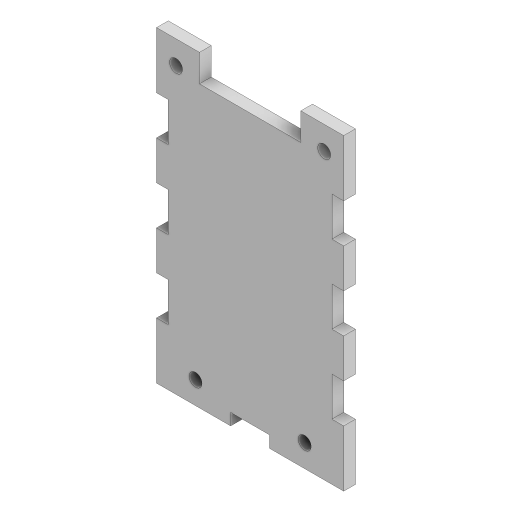
# Autodesk Inventor part: Bottom piece
Saved by Autodesk Inventor 2023.3 (Build 273359000, 359)
## iProperties
Created: 2024-09-20
Part Number: Bottom piece
Material: Generic
Document SubType Name: Modeling
Designer: David Zindović
Density: 1 g/cm^3
Appearance: Default
Author: David Zindović
Autodesk Inventor part; units mm, degrees
ref_plane "YZ Plane" through (0, 0, 0) normal (1, 0, 0) x (0, 1, 0)
ref_plane "XZ Plane" through (0, 0, 0) normal (0, 1, 0) x (-1, 0, 0)
ref_plane "XY Plane" through (0, 0, 0) normal (0, 0, 1) x (1, 0, 0)
sketch "Sketch1" plane through (0, 0, 0) normal (0, 0, 1) x (1, 0, 0)
  circle A0 centre (-22.4743, -28.7795) radius 1.65
  circle A1 centre (5.5257, -28.7795) radius 1.65
  circle A2 centre (-27.4743, 38.4705) radius 1.65
  circle A3 centre (10.5257, 38.4705) radius 1.65
  line L0 (-25.4743, 18.4705) -> (8.5257, 18.4705)
  line L1 (8.5257, 18.4705) -> (8.5257, -25.5295)
  line L2 (8.5257, -25.5295) -> (-25.4743, -25.5295)
  line L3 (-25.4743, -25.5295) -> (-25.4743, 18.4705)
  circle A4 centre (-8.4743, 28.4705) radius 2.5
  line L4 (-32.4743, 44.4705) -> (15.5257, 44.4705)
  line L5 (15.5257, 44.4705) -> (15.5257, -34.5295)
  line L6 (15.5257, -34.5295) -> (-32.4743, -34.5295)
  line L7 (-32.4743, -34.5295) -> (-32.4743, 44.4705)
  line L8 (-25.4743, -25.5295) -> (8.5257, -25.5295)
  line L9 (8.5257, -25.5295) -> (8.5257, -26.5295)
  line L10 (8.5257, -26.5295) -> (-25.4743, -26.5295)
  line L11 (-25.4743, -26.5295) -> (-25.4743, -25.5295)
  line L12 (-24.1243, -28.7795) -> (-24.1243, -26.5295)
  line L13 (-20.8243, -28.7795) -> (-20.8243, -26.5295)
  line L14 (3.8757, -28.7795) -> (3.8757, -26.5295)
  line L15 (7.1757, -28.7795) -> (7.1757, -26.5295)
  line L16 (-32.4743, 9.9705) -> (-29.4743, 9.9705)
  line L17 (-29.4743, 9.9705) -> (-29.4743, -0.0295)
  line L18 (-29.4743, -0.0295) -> (-32.4743, -0.0295)
  line L19 (-32.4743, -0.0295) -> (-32.4743, 9.9705)
  line L20 (-13.4743, -34.5295) -> (-3.4743, -34.5295)
  line L21 (-3.4743, -34.5295) -> (-3.4743, -31.5295)
  line L22 (-3.4743, -31.5295) -> (-13.4743, -31.5295)
  line L23 (-13.4743, -31.5295) -> (-13.4743, -34.5295)
  line L24 (-13.4743, 44.4705) -> (-3.4743, 44.4705)
  line L25 (-3.4743, 44.4705) -> (-3.4743, 41.4705)
  line L26 (-3.4743, 41.4705) -> (-13.4743, 41.4705)
  line L27 (-13.4743, 41.4705) -> (-13.4743, 44.4705)
  line L28 (-29.4743, 29.9705) -> (-29.4743, 19.9705)
  line L29 (-29.4743, 19.9705) -> (-32.4743, 19.9705)
  line L30 (-32.4743, 29.9705) -> (-29.4743, 29.9705)
  line L31 (-29.4743, -20.0295) -> (-32.4743, -20.0295)
  line L32 (-29.4743, -10.0295) -> (-29.4743, -20.0295)
  line L33 (-32.4743, -10.0295) -> (-29.4743, -10.0295)
  line L34 (12.5257, 9.9705) -> (15.5257, 9.9705)
  line L35 (15.5257, 9.9705) -> (15.5257, -0.0295)
  line L36 (15.5257, -0.0295) -> (12.5257, -0.0295)
  line L37 (12.5257, -0.0295) -> (12.5257, 9.9705)
  line L38 (15.5257, -20.0295) -> (12.5257, -20.0295)
  line L39 (12.5257, -20.0295) -> (12.5257, -10.0295)
  line L40 (12.5257, -10.0295) -> (15.5257, -10.0295)
  line L41 (15.5257, 19.9705) -> (12.5257, 19.9705)
  line L42 (12.5257, 19.9705) -> (12.5257, 29.9705)
  line L43 (12.5257, 29.9705) -> (15.5257, 29.9705)
  line L44 (-21.4743, 44.4705) -> (4.5257, 44.4705)
  line L45 (4.5257, 44.4705) -> (4.5257, 37.4705)
  line L46 (4.5257, 37.4705) -> (-21.4743, 37.4705)
  line L47 (-21.4743, 37.4705) -> (-21.4743, 44.4705)
  point P0 (0, 0)
  point P1 (-8.4743, -3.5295)
  point P2 (-8.4743, 18.4705)
  point P3 (-8.4743, -25.5295)
  point P4 (8.5257, -3.5295)
  point P5 (-8.4743, 44.4705)
  point P6 (-32.4743, 4.9705)
  point P7 (-8.4743, -31.5295)
  point P8 (-8.4743, -34.5295)
  point P9 (-8.4743, -34.5295)
  point P10 (-8.4743, 41.4705)
  point P11 (15.5257, 4.9705)
  point P12 (15.5257, 4.9705)
  point P13 (-8.4743, 37.4705)
  point P14 (-8.4743, 44.4705)
  dimension "d16" = 3.3
  dimension "d17" = 3.3
  dimension "d18" = 28
  dimension "d19" = 14
  dimension "d20" = 3.3
  dimension "d21" = 3.3
  dimension "d22" = 38
  dimension "d23" = 19
  dimension "d24" = 34
  dimension "d25" = 44
  dimension "d26" = 3.25
  dimension "d27" = 20
  dimension "d28" = 5
  dimension "d29" = 10
  dimension "d30" = 9
  dimension "d31" = 26
  dimension "d32" = 7
  dimension "d33" = 1
  dimension "d34" = 3
  dimension "d35" = 10
  dimension "d36" = 10
  dimension "d37" = 3
  dimension "d38" = 10
  dimension "d39" = 3
  dimension "d40" = 20
  dimension "d41" = 20
  dimension "d42" = 3
  dimension "d43" = 10
  dimension "d44" = 20
  dimension "d45" = 20
  dimension "d52" = 26
  dimension "d53" = 7
  constraints: 96 end point, 16 parallel, 14 midpoint, 11 perpendicular, 8 horizontal, 8 vertical alignment, 7 point on line, 5 centre point, 5 vertical, 4 point on circle, 4 tangent, 3 horizontal alignment, 1 coincident, 1 collinear, 28 other
  measures "d16" diameter of A0
  measures "d17" diameter of A1
  measures "d18" distance of A1.centre A0.centre
  measures "d19" horizontal distance of point (-8.474, -3.529) A0.centre
  measures "d20" diameter of A2
  measures "d21" diameter of A3
  measures "d22" distance of A3.centre A2.centre
  measures "d23" horizontal distance of point (-8.474, -3.529) A2.centre
  measures "d24" distance of L1.end L2.end
  measures "d25" distance of L0.end L1.end
  measures "d26" distance from line of L2 A1.centre
  measures "d27" distance from line of L0 A2.centre
  measures "d28" diameter of A4
  measures "d29" distance from line of L0 A4.centre
  measures "d30" distance between parallel lines of L2 L6
  measures "d31" distance between parallel lines of L4 L0
  measures "d32" distance between parallel lines of L5 L1
  measures "d33" distance of L8.end L9.end
  measures "d34" distance of L17.end L18.end
  measures "d35" distance of L16.end L17.end
  measures "d36" distance of L21.end L22.end
  measures "d37" distance of L20.end L21.end
  measures "d38" distance of L25.end L26.end
  measures "d39" distance of L24.end L25.end
  measures "d40" distance of L16.end L28.start
  measures "d41" distance of L17.end L31.start
  measures "d42" distance of L35.end L36.end
  measures "d43" distance of L34.end L35.end
  measures "d44" distance of L36.end L38.end
  measures "d45" distance of L36.end L41.end
  measures "d52" distance of L45.end L46.end
  measures "d53" distance of L46.end L44.start
extrude "Extrusion1" add sketch "Sketch1" along normal mid plane 3 contours A0 L12 L10 L13 | L10 L11 L2 L9 | L10 L15 A1 L14 | L3 L0 L1 L2 | A4 | L4 L47 L46 L45 L5 L43 L42 L41 L34 L37 L36 L40 L39 L38 L6 L21 L22 L23 L7 L31 L32 L33 L18 L17 L16 L29 L28 L30
equation "\"d19\" = 0.5 * d18"
equation "\"d23\" = 0.5 * d22"
body "Solid1"
